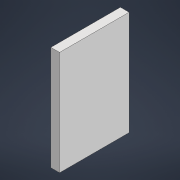
# Autodesk Inventor part: Общий концепт в 3д
Saved by Autodesk Inventor 2022 (Build 260153000, 153)
## iProperties
Created: 2023-02-10
Part Number: Общий концепт в 3д
Material: Типовые
Document SubType Name: Modeling
Designer: Глеб
Density: 1 g/cm^3
Appearance: По умолчанию
Mass: 12000 g
Surface Area: 5800 cm^2
Volume: 12000 cm^3
Author: Глеб
Autodesk Inventor part; units mm, degrees
ref_plane "YZ Plane" through (0, 0, 0) normal (1, 0, 0) x (0, 1, 0)
ref_plane "XZ Plane" through (0, 0, 0) normal (0, 1, 0) x (-1, 0, 0)
ref_plane "XY Plane" through (0, 0, 0) normal (0, 0, 1) x (1, 0, 0)
sketch "Эскиз1" plane through (0, 0, 0) normal (1, 0, 0) x (0, 1, 0)
  line L0 (-270, 200) -> (330, 200)
  line L1 (330, 200) -> (330, -200)
  line L2 (330, -200) -> (-270, -200)
  line L3 (-270, -200) -> (-270, 200)
  line L4 (-270, 200) -> (330, -200) construction
  line L5 (330, 200) -> (-270, -200) construction
  point P0 (30, 0)
  point P1 (0, 0)
  dimension "d0" = 400
  dimension "d1" = 600
  dimension "d73" = 30
  constraints: 12 end point, 2 midpoint, 2 parallel, 1 horizontal, 1 perpendicular
  measures "d0" distance of L0.end L1.end
  measures "d1" distance of L1.end L2.end
  measures "d73" distance of point (30, 0) point (0, 0)
extrude "Выдавливание1" add sketch "Эскиз1" along normal blind 50
